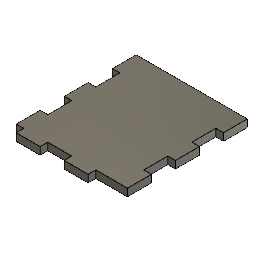
Top (Autodesk Fusion 360 design; units mm, degrees)
Autodesk Fusion 360 part; units mm, degrees
sketch "Sketch1" plane through (0, 0, 0) normal (0, 1, 0) x (1, 0, 0)
  line L0 (80, 100) -> (0, 100)
  line L1 (20, 0) -> (20, -6.35)
  line L2 (20, -6.35) -> (0, -6.35)
  line L3 (0, -6.35) -> (0, 0)
  line L4 (60, 0) -> (60, -6.35)
  line L5 (60, -6.35) -> (40, -6.35)
  line L6 (40, -6.35) -> (40, 0)
  line L7 (0, 0) -> (-6.35, 0)
  line L8 (-6.35, 0) -> (-6.35, 20)
  line L9 (-6.35, 20) -> (0, 20)
  line L10 (0, 40) -> (-6.35, 40)
  line L11 (-6.35, 40) -> (-6.35, 60)
  line L12 (-6.35, 60) -> (0, 60)
  line L13 (0, 80) -> (-6.35, 80)
  line L14 (-6.35, 80) -> (-6.35, 100)
  line L15 (-6.35, 100) -> (0, 100)
  line L16 (80, 0) -> (86.35, 0)
  line L17 (86.35, 0) -> (86.35, 20)
  line L18 (86.35, 20) -> (80, 20)
  line L19 (80, 60) -> (86.35, 60)
  line L20 (86.35, 60) -> (86.35, 40)
  line L21 (86.35, 40) -> (80, 40)
  line L22 (80, 100) -> (86.35, 100)
  line L23 (86.35, 100) -> (86.35, 80)
  line L24 (86.35, 80) -> (80, 80)
  line L25 (0, 20) -> (-6.35, 20)
  line L26 (-6.35, 20) -> (-6.35, 0)
  line L27 (-6.35, 0) -> (0, 0)
  line L28 (0, 0) -> (0, -6.35)
  line L29 (0, -6.35) -> (20, -6.35)
  line L30 (20, -6.35) -> (20, -1.6258)
  line L31 (20, -6.35) -> (20, 0)
  line L32 (20, 0) -> (40, 0)
  line L33 (40, 0) -> (40, -6.35)
  line L34 (40, -6.35) -> (60, -6.35)
  line L35 (60, -6.35) -> (60, 0)
  line L36 (60, 0) -> (86.35, 0)
  line L37 (86.35, 0) -> (86.35, 20)
  line L38 (86.35, 20) -> (80, 20)
  line L39 (80, 20) -> (80, 40)
  line L40 (80, 40) -> (86.35, 40)
  line L41 (86.35, 40) -> (86.35, 60)
  line L42 (86.35, 60) -> (80, 60)
  line L43 (80, 60) -> (80, 80)
  line L44 (80, 80) -> (86.35, 80)
  line L45 (86.35, 80) -> (86.35, 100)
  line L46 (86.35, 100) -> (-6.35, 100)
  line L47 (-6.35, 100) -> (-6.35, 80)
  line L48 (-6.35, 80) -> (0, 80)
  line L49 (0, 80) -> (0, 60)
  line L50 (0, 60) -> (-6.35, 60)
  line L51 (-6.35, 60) -> (-6.35, 40)
  line L52 (-6.35, 40) -> (0, 40)
  line L53 (0, 40) -> (0, 20)
  line L54 (0, 20) -> (-6.35, 20)
  line L55 (-6.35, 20) -> (-6.35, 0)
  line L56 (-6.35, 0) -> (0, 0)
  dimension "d1" = 100
  dimension "d2" = 80
  dimension "d5" = 20
  dimension "d6" = 6.35
  dimension "d7" = 6.35
  dimension "d8" = 20
  dimension "d9" = 20
  dimension "d10" = 6.35
  dimension "d11" = 20
  dimension "d12" = 6.35
  dimension "d13" = 20
  dimension "d14" = 20
  dimension "d15" = 6.35
  dimension "d16" = 20
  dimension "d17" = 20
  dimension "d18" = 6.35
  dimension "d19" = 20
  dimension "d20" = 6.35
  dimension "d21" = 20
  dimension "d22" = 20
  dimension "d23" = 6.35
  dimension "d24" = 20
  measures "d1" distance of L3.end
  measures "d2" distance of L3.end
  measures "d6" distance of L3.end
  measures "d9" distance of L1 L6
  measures "d10" distance of L3.end
  measures "d14" distance of L9 L10
  measures "d17" distance of L12 L13
  measures "d19" distance of L3.end
extrude "Extrude3" add sketch "Sketch1" along normal blind 6.35
extrude "Extrude2" [suppressed]
extrude "Extrude1" [suppressed]
